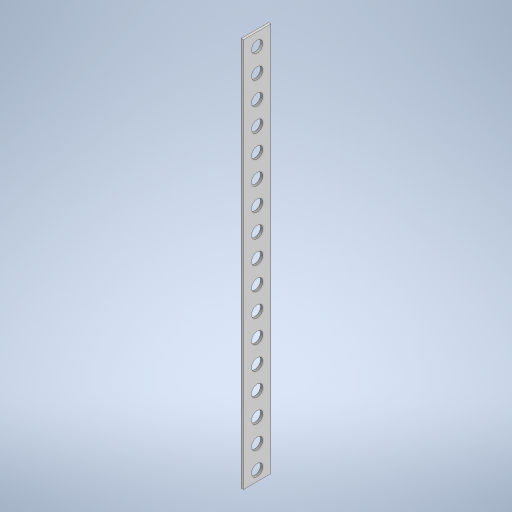
# Autodesk Inventor part: aste2
Saved by Autodesk Inventor 2023 (Build 270158000, 158)
## iProperties
Created: 2023-08-10
Part Number: aste2
Material: Genérico
Document SubType Name: Modeling
Designer: azeve
Density: 1 g/cm^3
Appearance: Padrão
Author: azeve
Autodesk Inventor part; units mm, degrees
ref_plane "YZ Plane" through (0, 0, 0) normal (1, 0, 0) x (0, 1, 0)
ref_plane "XZ Plane" through (0, 0, 0) normal (0, 1, 0) x (-1, 0, 0)
ref_plane "XY Plane" through (0, 0, 0) normal (0, 0, 1) x (1, 0, 0)
sketch "Esboço1" plane through (0, 0, 0) normal (1, 0, 0) x (0, 1, 0)
  line L0 (19.0364, -63.7913) -> (-150.9636, -63.7913)
  line L1 (-150.9636, -63.7913) -> (-150.9636, -51.7913)
  line L2 (19.0364, -51.7913) -> (19.0364, -63.7913)
  circle A0 centre (-146.5949, -57.7913) radius 2.5
  line L3 (19.0364, -51.7913) -> (-150.9636, -51.7913)
  circle A1 centre (-136.5949, -57.7913) radius 2.5
  circle A2 centre (-126.5949, -57.7913) radius 2.5
  circle A3 centre (-116.5949, -57.7913) radius 2.5
  circle A4 centre (-106.5949, -57.7913) radius 2.5
  circle A5 centre (-96.5949, -57.7913) radius 2.5
  circle A6 centre (-86.5949, -57.7913) radius 2.5
  circle A7 centre (-76.5949, -57.7913) radius 2.5
  circle A8 centre (-66.5949, -57.7913) radius 2.5
  circle A9 centre (-56.5949, -57.7913) radius 2.5
  circle A10 centre (-46.5949, -57.7913) radius 2.5
  circle A11 centre (-36.5949, -57.7913) radius 2.5
  circle A12 centre (-26.5949, -57.7913) radius 2.5
  circle A13 centre (-16.5949, -57.7913) radius 2.5
  circle A14 centre (-6.5949, -57.7913) radius 2.5
  circle A15 centre (3.4051, -57.7913) radius 2.5
  circle A16 centre (13.4051, -57.7913) radius 2.5
  point P0 (0, 0)
  dimension "d2" = 12
  dimension "d3" = 170
  dimension "d4" = 5
  dimension "d10" = 10
  constraints: 17 centre point, 8 end point, 3 horizontal, 1 perpendicular, 1 vertical, 32 other
  measures "d2" distance of L0.end L1.end
  measures "d3" distance of L0.start L0.end
  measures "d4" diameter of A0
  measures "d10" distance of A0.centre A1.centre
extrude "Extrusão1" add sketch "Esboço1" along normal blind 1
